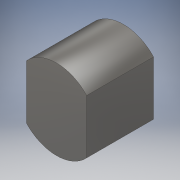
# Autodesk Inventor part: Motor
Saved by Autodesk Inventor 2018 (Build 220112000, 112)
## iProperties
Created: 2018-01-12
Part Number: Motor
Material: Stainless Steel
Document SubType Name: Modeling
Designer: Kyle
Density: 8 g/cm^3
Appearance: Semi-Polished
Author: Kyle
Autodesk Inventor part; units mm, degrees
ref_plane "YZ Plane" through (0, 0, 0) normal (1, 0, 0) x (0, 1, 0)
ref_plane "XZ Plane" through (0, 0, 0) normal (0, 1, 0) x (-1, 0, 0)
ref_plane "XY Plane" through (0, 0, 0) normal (0, 0, 1) x (1, 0, 0)
sketch "Sketch1" plane through (0, 0, 0) normal (0, 0, 1) x (1, 0, 0)
  line L0 (0, 0) -> (0, -13.335)
  line L1 (14.859, 0) -> (14.859, -13.335)
  arc A0 (14.859, 0) -> (0, 0) centre (7.4295, -6.9028) ccw
  arc A1 (0, -13.335) -> (14.859, -13.335) centre (7.4295, -6.4322) ccw
  point P0 (7.4295, 3.2385)
  point P1 (7.4295, -16.5735)
  dimension "d0" = 14.859
  dimension "d1" = 13.335
  dimension "d2" = 3.2385
  dimension "d3" = 7.4295
  dimension "d4" = 3.2385
  constraints: 6 point on circle, 4 end point, 2 centre point, 2 vertical, 1 coincident
  measures "d0" distance of L0.start L1.start
  measures "d1" distance of L0.end L0.start
  measures "d2" vertical distance of L0.start point (7.429, 3.239)
  measures "d3" horizontal distance of point (0, 0) point (7.429, 3.239)
  measures "d4" vertical distance of L0.end point (7.429, -16.574)
extrude "Extrusion1" add sketch "Sketch1" along normal blind 16.51
body "Solid1"
